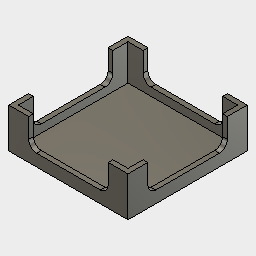
Breadboard Mount v3 (Autodesk Fusion 360 design; units mm, degrees)
Autodesk Fusion 360 part; units mm, degrees
sketch "Sketch5" plane through (0, 0, 0) normal (0, 1, 0) x (1, 0, 0)
  line L0 (0, 0) -> (30, 0)
  line L1 (30, 0) -> (30, -30)
  line L2 (30, -30) -> (0, -30)
  line L3 (0, -30) -> (0, 0)
  dimension "d48" = 30
  dimension "d49" = 30
  constraint horizontal L0
  constraint vertical L1
  constraint horizontal L2
  constraint vertical L3
  constraint coincident L0.start L3.end
extrude "Extrude4" add sketch "Sketch5" along normal blind 1
sketch "Sketch6" plane through (0, 1, 0) normal (0, 1, 0) x (-1, 0, 0)
  line L0 (0, 30) -> (-30, 30)
  line L1 (-30, 30) -> (-30, 0)
  line L2 (-30, 0) -> (0, 0)
  line L3 (0, 0) -> (0, 30)
  line L4 (-1.2, 28.8) -> (-28.8, 28.8)
  line L5 (-28.8, 28.8) -> (-28.8, 1.2)
  line L6 (-28.8, 1.2) -> (-1.2, 1.2)
  line L7 (-1.2, 1.2) -> (-1.2, 28.8)
  dimension "d52" = 1.2
extrude "Extrude5" add sketch "Sketch6" along normal blind 2
sketch "Sketch7" plane through (0, 3, 0) normal (0, 1, 0) x (-1, 0, 0)
  line L0 (-1.2, 28.8) -> (-1.2, 1.2)
  line L1 (-1.2, 1.2) -> (-28.8, 1.2)
  line L2 (-28.8, 1.2) -> (-28.8, 28.8)
  line L3 (-28.8, 28.8) -> (-1.2, 28.8)
  line L4 (0, 0) -> (0, 30)
  line L5 (0, 30) -> (-30, 30)
  line L6 (-30, 30) -> (-30, 0)
  line L7 (-30, 0) -> (0, 0)
  line L8 (0, 0) -> (0, 5)
  line L9 (0, 5) -> (-1.2001, 5)
  line L10 (-1.2001, 5) -> (-1.2, 1.2)
  line L11 (-1.2, 1.2) -> (-5, 1.2)
  line L12 (-5, 1.2) -> (-5, -0.0001)
  line L13 (-5, -0.0001) -> (0, 0)
  line L14 (0, 30) -> (0, 25)
  line L15 (-5, 30.0001) -> (0, 30)
  line L16 (-1.2, 28.8) -> (-5, 28.8)
  line L17 (-1.2001, 25) -> (-1.2, 28.8)
  line L18 (0, 25) -> (-1.2001, 25)
  line L19 (-5, 28.8) -> (-5, 30.0001)
  line L20 (-28.7999, 5) -> (-28.8, 1.2)
  line L21 (-30, 0) -> (-30, 5)
  line L22 (-30, 5) -> (-28.7999, 5)
  line L23 (-28.8, 1.2) -> (-25, 1.2)
  line L24 (-25, 1.2) -> (-25, -0.0001)
  line L25 (-25, -0.0001) -> (-30, 0)
  line L26 (-30, 25) -> (-28.7999, 25)
  line L27 (-30, 30) -> (-30, 25)
  line L28 (-28.7999, 25) -> (-28.8, 28.8)
  line L29 (-28.8, 28.8) -> (-25, 28.8)
  line L30 (-25, 28.8) -> (-25, 30.0001)
  line L31 (-25, 30.0001) -> (-30, 30)
  dimension "d55" = 5
  dimension "d56" = 1.2001
  dimension "d57" = 3.8
  dimension "d58" = 1.2001
  constraint coincident L4.start L7.end
  constraint vertical L8
  constraint horizontal L9
  constraint horizontal L11
  constraint vertical L12
extrude "Extrude6" add sketch "Sketch7" along normal blind 7 contours L0 L3 L4 L5 L14 L15 L16 L17 L18 L19 | L0 L1 L4 L7 L8 L9 L10 L11 L12 L13 | L2 L3 L5 L6 L26 L27 L28 L29 L30 L31 | L1 L2 L6 L7 L20 L21 L22 L23 L24 L25
fillet "Fillet5" radius 2 8 edges at (0.6, 3, 5) (0.6, 3, 25) (5, 3, 29.4) (25, 3, 29.4) (29.4, 3, 5) (25, 3, 0.6) (5, 3, 0.6) (29.4, 3, 25)
